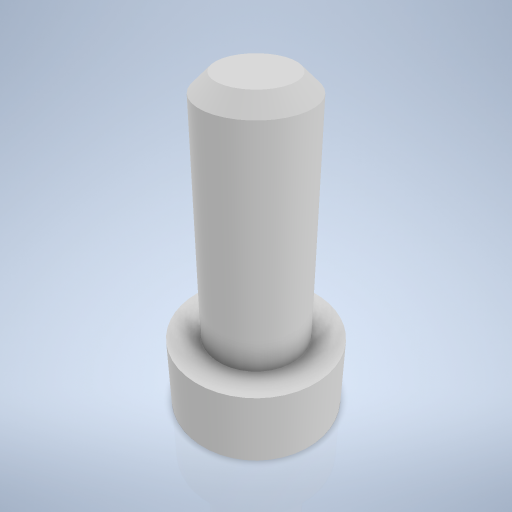
# Autodesk Inventor part: bolt_shaft
Saved by Autodesk Inventor 2024.2 (Build 282272000, 272)
## iProperties
Created: 2024-05-17
Part Number: bolt_shaft
Material: Generisch
Document SubType Name: Modeling
Designer: Fabri
Density: 1 g/cm^3
Appearance: Vorgabe
Author: Fabri
Autodesk Inventor part; units mm, degrees
ref_plane "YZ Plane" through (0, 0, 0) normal (1, 0, 0) x (0, 1, 0)
ref_plane "XZ Plane" through (0, 0, 0) normal (0, 1, 0) x (-1, 0, 0)
ref_plane "XY Plane" through (0, 0, 0) normal (0, 0, 1) x (1, 0, 0)
sketch "Skizze1" plane through (0, 0, 0) normal (0, 1, 0) x (-1, 0, 0)
  line L0 (0, 0) -> (3.25, 0)
  line L1 (3.25, 0) -> (3.25, -16)
  line L2 (3.25, -16) -> (5.25, -16)
  line L3 (5.25, -16) -> (5.25, -21)
  line L4 (5.25, -21) -> (0, -21)
  line L5 (0, -21) -> (0, 0)
  dimension "d0" = 6.5
  dimension "d1" = 10.5
  dimension "d2" = 21
  dimension "d3" = 16
  constraints: 12 end point, 5 perpendicular, 1 horizontal
  measures "d0" diameter of L1 L5
  measures "d1" diameter of L3 L5
  measures "d2" distance between parallel lines of L4 L0
  measures "d3" distance between parallel lines of L0 L2
revolve "Umdrehung1" add sketch "Skizze1" angle 360 about axis through (0, 0, -21) along (0, 0, 1)
chamfer "Fasen1" distance 1 angle 45 1 edges at (3.25, 0, 0)
